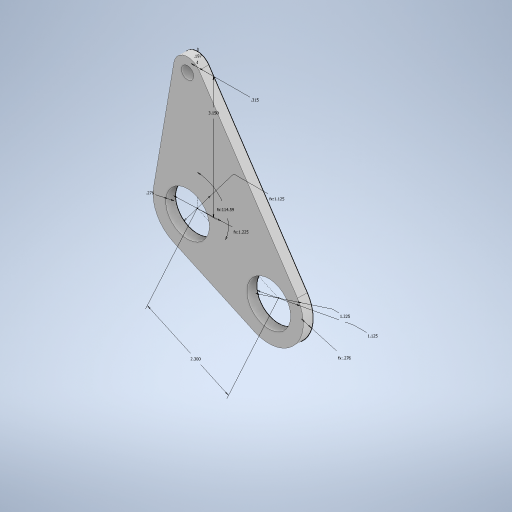
# Autodesk Inventor part: sussy pivot
Saved by Autodesk Inventor 2023 (Build 270158000, 158)
## iProperties
Created: 2022-04-01
Part Number: sussy pivot
Material: Generic
Document SubType Name: Modeling
Designer: Zain Ali
Density: 1 g/cm^3
Appearance: Default
Author: Zain Ali
Autodesk Inventor part; units mm, degrees
ref_plane "YZ Plane" through (0, 0, 0) normal (1, 0, 0) x (0, 1, 0)
ref_plane "XZ Plane" through (0, 0, 0) normal (0, 1, 0) x (-1, 0, 0)
ref_plane "XY Plane" through (0, 0, 0) normal (0, 0, 1) x (1, 0, 0)
sketch "Sketch1" plane through (0, 0, 0) normal (0, 0, 1) x (1, 0, 0)
  circle A0 centre (0, 0) radius 14.2875
  circle A1 centre (53.1212, -24.3113) radius 14.2875
  circle A2 centre (0, 80) radius 4
  line L0 (0, 80) -> (0, 0) construction
  line L1 (0, 0) -> (53.1212, -24.3113) construction
  circle A3 centre (53.1212, -24.3113) radius 15.5575
  circle A4 centre (0, 0) radius 15.5575
  arc A5 (43.7339, -44.8228) -> (71.9014, -11.8155) centre (53.1212, -24.3113) ccw
  arc A6 (-22.2312, 3.8228) -> (-9.3872, -20.5115) centre (0, 0) ccw
  arc A7 (7.4929, 84.9856) -> (-8.8698, 81.5252) centre (0, 80) ccw
  line L2 (-8.8698, 81.5252) -> (-22.2312, 3.8228)
  line L3 (-9.3872, -20.5115) -> (43.7339, -44.8228)
  line L4 (71.9014, -11.8155) -> (7.4929, 84.9856)
  dimension "d0" = 8
  dimension "d1" = 28.575
  dimension "d4" = 28.575
  dimension "d5" = 58.42
  dimension "d6" = 114.592
  dimension "d7" = 80
  dimension "d8" = 31.115
  dimension "d9" = 31.115
  dimension "d10" = 5
  dimension "d11" = 7
  dimension "d13" = 7
  constraints: 10 end point, 8 centre point, 7 coincident, 6 point on circle, 6 tangent, 1 vertical
  measures "d0" diameter of A2
  measures "d1" diameter of A1
  measures "d4" diameter of A0
  measures "d5" distance of L1.end L0.end
  measures "d6" angle of L1 L0
  measures "d7" distance of L0.start L0.end
  measures "d8" diameter of A3
  measures "d9" diameter of A4
  measures "d10" radial gap between concentric circles of A7 A2
  measures "d11" radial gap between concentric circles of A6 A4
  measures "d13" radial gap between concentric circles of A5 A3
extrude "Extrusion1" add sketch "Sketch1" along normal blind 6.35 contours A3 | A4 | L3 A6 L2 A7 L4 A5
equation "\"d4\" = d1"
equation "\"d6\" = d2"
equation "\"d9\" = d8"
equation "\"d13\" = d11"
equation "\"d2\" = 114.591559deg"
body "Solid1"
